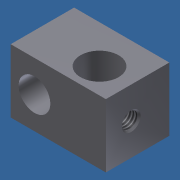
# Autodesk Inventor part: MANCAL DO EIXO DIANTEIRO(7)
Saved by Autodesk Inventor 2012 SP2 (Build 160219200, 219)
## iProperties
Created: 2012-07-23
Part Number: MANCAL DO EIXO DIANTEIRO(7)
Material: Carbon Steel
Document SubType Name: Modeling
Designer: bruno.silveira
Mass: 94.44 g
Surface Area: 32 cm^2
Volume: 12 cm^3
Density: 7.87 g/cm^3
Author: bruno.silveira
Autodesk Inventor part; units mm, degrees
ref_plane "YZ Plane" through (0, 0, 0) normal (1, 0, 0) x (0, 1, 0)
ref_plane "XZ Plane" through (0, 0, 0) normal (0, 1, 0) x (-1, 0, 0)
ref_plane "XY Plane" through (0, 0, 0) normal (0, 0, 1) x (1, 0, 0)
sketch "Sketch1" plane through (0, 0, 0) normal (0, 0, 1) x (1, 0, 0)
  line L0 (0, 0) -> (30, 0)
  line L1 (30, 0) -> (30, 20)
  line L2 (30, 20) -> (0, 20)
  line L3 (0, 20) -> (0, 0)
  dimension "d0" = 30
  dimension "d1" = 20
  constraints: 8 end point, 2 parallel, 1 horizontal, 1 perpendicular
  measures "d0" distance of L1.end L2.end
  measures "d1" distance of L2.end L0.start
extrude "Extrusion1" add sketch "Sketch1" along normal blind 20
sketch "Sketch2" plane through (0, 0, 0) normal (0, -1, 0) x (1, 0, 0)
  line L0 (30, 20) -> (0, 20) projected
  line L1 (0, 0) -> (0, 20) projected
  point P0 (7.5, 10)
  dimension "d4" = 7.5
  dimension "d5" = 10
  measures "d4" distance from line of L1 point (7.5, 10)
  measures "d5" distance from line of L0 point (7.5, 10)
hole "Hole1" at (7.5, 0, 10) direction (0, 1, 0) diameter 6.5 depth 20 tip angle 118 counterbore diameter 10 counterbore depth 13
sketch "Sketch3" plane through (0, 0, 20) normal (0, 0, 1) x (1, 0, 0)
  line L0 (0, 0) -> (0, 20) projected
  line L1 (0, 20) -> (30, 20) projected
  point P0 (20, 8)
  dimension "d13" = 20
  dimension "d14" = 12
  measures "d13" distance from line of L0 point (20, 8)
  measures "d14" distance from line of L1 point (20, 8)
hole "Hole2" at (20, 8, 20) direction (0, 0, -1) diameter 12 depth 20 tip angle 118
sketch "Sketch4" plane through (30, 0, 0) normal (1, 0, 0) x (0, 0, -1)
  line L0 (0, 0) -> (0, 20) projected
  line L1 (0, 20) -> (-20, 20) projected
  point P0 (-10, 8)
  dimension "d22" = 10
  dimension "d23" = 12
  measures "d22" distance from line of L0 point (-10, 8)
  measures "d23" distance from line of L1 point (-10, 8)
hole "Hole3" at (30, 8, 10) direction (-1, 0, 0) diameter 4.917 depth 6 tip angle 118 thread size "M6x1" class "6H" standard "ANSI Metric M Profile"
chamfer "Chamfer1" distance 0.5 angle 45 1 edges at (30, 8, 12.4585)
equation "\"d17\" = d14"
equation "\"d26\" = d14"
body "Solid1"
